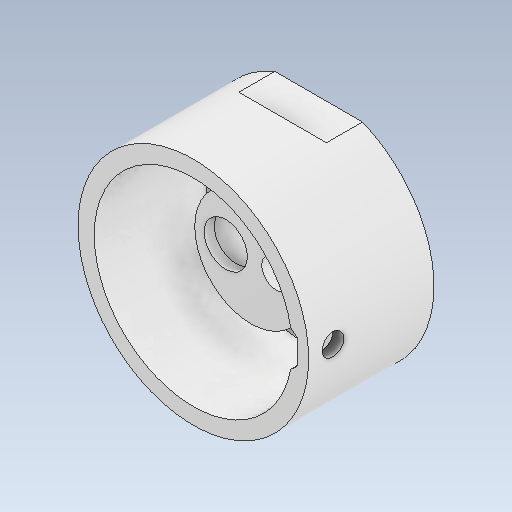
# Autodesk Inventor part: Bottom
Saved by Autodesk Inventor 2020.2 (Build 242310000, 310)
## iProperties
Created: 2021-08-11
Part Number: Bottom
Material: PC/ABS-Kunststoff
Document SubType Name: Modeling
Designer: johan
Density: 0.357273 g/cm^3
Appearance: Glatt - Weiß
Author: johan
Autodesk Inventor part; units mm, degrees
ref_plane "XZ Plane" through (0, 0, 0) normal (0, 1, 0) x (-1, 0, 0)
sketch "Skizze1" plane through (0, 0, 0) normal (0, 0, 1) x (1, 0, 0)
  circle A0 centre (0, 0) radius 16
  circle A1 centre (-3.5, 0) radius 3
  circle A2 centre (3.5, 0) radius 2
  line L0 (-22.4, 0) -> (22.4, 0) construction
  line L1 (0, -22.4) -> (0, 22.4) construction
  circle A3 centre (0, 0) radius 3.5 construction
  dimension "d0" = 32
  dimension "d3" = 6
  dimension "d4" = 4
  dimension "d5" = 3.5
  dimension "d6" = 3.5
  dimension "d7" = 7
  constraints: 3 centre point, 2 coincident, 1 horizontal alignment, 1 point on line, 2 other
  measures "d0" diameter of A0
  measures "d3" diameter of A1
  measures "d4" diameter of A2
  measures "d5" distance of point (0, 0) A2.centre
  measures "d6" distance of point (0, 0) A1.centre
  measures "d7" distance of A2.centre A1.centre
extrude "Extrusion1" add sketch "Skizze1" along normal blind 3.6
sketch "Skizze2" plane through (0, 0, 3.6) normal (0, 0, 1) x (1, 0, 0)
  circle A0 centre (0, 0) radius 16
  circle A1 centre (-3.5, 0) radius 3 projected
  circle A2 centre (-3.5, 0) radius 3
  circle A3 centre (3.5, 0) radius 2 projected
  circle A4 centre (3.5, 0) radius 2
  circle A5 centre (0, 0) radius 7.8
  circle A6 centre (0, 0) radius 13.75
  dimension "d10" = 15.6
  dimension "d11" = 27.5
  dimension "d12" = 4
  dimension "d13" = 32
  dimension "d14" = 6
  constraints: 5 centre point, 5 coincident
  measures "d10" diameter of A5
  measures "d11" diameter of A6
  measures "d12" diameter of A4
  measures "d13" diameter of A0
  measures "d14" diameter of A2
extrude "Extrusion2" add sketch "Skizze2" along normal blind 5.8
sketch "Skizze4" plane through (0, 0, 0) normal (0, 0, -1) x (-1, 0, 0)
  circle A0 centre (0, 0) radius 7.8 construction
  circle A1 centre (3.5, 0) radius 3 construction
  circle A2 centre (-3.5, 0) radius 2 construction
  circle A3 centre (0, 0) radius 7
  dimension "d29" = 14
  constraints: 1 centre point, 1 coincident
  measures "d29" diameter of A3
extrude "Extrusion4" cut sketch "Skizze4" against normal blind 8
sketch "Skizze5" plane through (0, 0, 8) normal (0, 0, -1) x (-1, 0, 0)
  circle A0 centre (-3.5, 0) radius 2 construction
  line L0 (-1.5, 0) -> (0.5, 0) construction
  circle A1 centre (3.5, 0) radius 3 construction
  line L1 (-0.5, -6.9821) -> (-0.5, 6.9821) construction
  circle A2 centre (0, 0) radius 7 construction
  circle A3 centre (0, 0) radius 7
  arc A4 (3.2508, 6.1994) -> (3.1701, -6.241) centre (7.631, -0.0495) ccw
  arc A5 (2.3003, 6.6112) -> (2.2144, -6.6405) centre (7.631, -0.0495) ccw
  point P0 (0.1, -6.9993)
  point P1 (0.1, 6.9993)
  point P2 (-1.1, -6.913)
  point P3 (-1.1, 6.913)
  dimension "d35" = 0
  dimension "d39" = 8.5312
  dimension "d40" = 7.6312
  dimension "d41" = 4
  dimension "d42" = 8.1311
  dimension "d43" = 0.0495
  dimension "d44" = 0.6
  dimension "d45" = 0.6
  dimension "d46" = 0.6
  dimension "d47" = 0.6
  constraints: 6 point on circle, 4 end point, 2 centre point, 2 horizontal alignment, 1 coincident, 1 horizontal, 1 vertical, 13 other
  measures "d35" distance from line of point (3.5, 0) L0
  measures "d39" radius of A5
  measures "d40" radius of A4
  measures "d41" distance from line of point (3.5, 0) L1
  measures "d42" distance from line of A4.centre L1
  measures "d43" distance from line of A4.centre L0
  measures "d44" distance from line of point (0.1, 6.999) L1
  measures "d45" distance from line of point (0.1, -6.999) L1
  measures "d46" distance from line of point (-1.1, 6.913) L1
  measures "d47" distance from line of point (-1.1, -6.913) L1
extrude "Extrusion5" add sketch "Skizze5" along normal blind 8 contours A4 A3 A5
sketch "Skizze6" plane through (0, 0, 3.6) normal (0, 0, 1) x (1, 0, 0)
  circle A0 centre (0, 0) radius 7.8 projected
  circle A1 centre (0, 0) radius 13.75 projected
extrude "Extrusion6" cut sketch "Skizze6" against normal blind 1.6
sketch "Skizze7" plane through (0, 0, 0) normal (0, 0, -1) x (-1, 0, 0)
  circle A0 centre (0, 0) radius 16 projected
  line L0 (0, 16) -> (0, 14.8) construction
  line L1 (0, 16) -> (1.2, 16) construction
  line L2 (0, 14.8) -> (-6.0795, 14.8)
  line L3 (0, 14.8) -> (6.0795, 14.8) construction
  line L4 (0, 14.8) -> (6.0795, 14.8)
  line L5 (0, 14.8) -> (6.0795, 14.8) construction
  point P0 (-0.8, 15.98)
  point P1 (0.8, 15.98)
  point P2 (0, 15.4)
  dimension "d50" = 1.2
  dimension "d51" = 90
  dimension "d70" = 1.18
  dimension "d71" = 1.18
  constraints: 14 end point, 4 point on circle, 3 equal length, 3 horizontal, 1 collinear, 1 midpoint, 1 parallel, 1 tangent, 1 vertical
  measures "d50" distance of L0.start L0.end
  measures "d51" angle of L0 L1
  measures "d70" distance from line of A0.end L5
  measures "d71" distance from line of point (-0.8, 15.98) L5
extrude "Extrusion7" cut sketch "Skizze7" against normal blind 5 contours L4 L2 A0 picked at (-3.0593, 15.099)
sketch "Skizze8" plane through (0, 0, 9.4) normal (0, 0, 1) x (1, 0, 0)
  circle A0 centre (0, 0) radius 13.75
  circle A1 centre (0, 0) radius 16
  dimension "d55" = 27.5
  dimension "d56" = 32
  constraints: 2 centre point, 2 coincident
  measures "d55" diameter of A0
  measures "d56" diameter of A1
extrude "Extrusion8" add sketch "Skizze8" along normal blind 8
ref_plane "Arbeitsebene1" through (16.5, 0, 0) normal (1, 0, 0) x (0, 1, 0)
sketch "Skizze9" plane through (16.5, 0, 0) normal (1, 0, 0) x (0, 1, 0)
  point P0 (0, 0)
  point P1 (0, 14)
  dimension "d67" = 14
  measures "d67" distance of point (0, 0) point (0, 14)
hole "Bohrung1" at (16.5, 0, 14) direction (-1, 0, 0) diameter 3 depth 3.25
sketch "Skizze10" plane through (0, 0, 0) normal (1, 0, 0) x (0, 1, 0)
  line L0 (14.8, 5) -> (14.8, 0) projected
  line L1 (14.8, 5) -> (16.0125, 6.2125)
  line L2 (14.8, 5) -> (16.5147, 5) construction
  line L3 (16.0125, 6.2125) -> (16.1276, 4.8849)
  line L4 (16.1276, 4.8849) -> (14.8, 5)
  point P0 (0, 0)
  dimension "d72" = 45
  dimension "d73" = 4.955
  dimension "d74" = 85.045
  dimension "d75" = 1.3127
  constraints: 8 end point, 1 equal length, 1 horizontal
  measures "d72" angle of L2 L1
  measures "d73" angle of L0 L3
  measures "d74" angle of L0 L4
  measures "d75" distance from line of L0.start L3
extrude "Extrusion9" cut sketch "Skizze10" against normal mid plane 29.25
ref_plane "Arbeitsebene2" through (0, 0, 13.9) normal (0, 0, 1) x (1, 0, 0)
sketch "Skizze11" plane through (0, 0, 13.9) normal (0, 0, 1) x (1, 0, 0)
  line L0 (13.6679, 1.5) -> (15.9295, 1.5) construction
  line L1 (13.6679, -1.5) -> (15.9295, -1.5) construction
  arc A0 (14.2726, -2.5) -> (14.2726, 2.5) centre (0, 0) ccw
  arc A1 (13.146, -2.5) -> (13.146, 2.5) centre (0, 0) ccw
  line L2 (14.2726, 2.5) -> (13.146, 2.5)
  line L3 (13.3816, 0) -> (15.9295, 0) construction
  line L4 (14.2726, -2.5) -> (13.146, -2.5)
  dimension "d79" = 14.4899
  dimension "d80" = 13.3816
  dimension "d81" = 4
  dimension "d82" = 1.5
  constraints: 6 end point, 5 point on circle, 2 centre point, 2 coincident, 2 symmetric about line, 1 horizontal, 1 parallel
  measures "d79" radius of A0
  measures "d80" radius of A1
  measures "d81" distance between parallel lines of L0 L4
  measures "d82" distance of L0.end L3.end
extrude "Extrusion10" cut sketch "Skizze11" along normal blind 3.75 and the other way blind 2
chamfer "Fase3" distance 0.6 angle 45 1 edges at (14.4899, 0, 11.9)
chamfer "Fase4" distance 0.1398 angle 45 2 edges at (13.6926, -1.2552, 11.9) (13.6926, 1.2552, 11.9)
chamfer "Fase5" distance 0.751 angle 45 2 edges at (14.2726, 2.5, 14.95) (14.2726, -2.5, 14.95)
